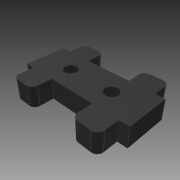
# Autodesk Inventor part: y_carriage_belt_iddler_holder
Saved by Autodesk Inventor 2014 (Build 180170000, 170)
## iProperties
Created: 2013-12-07
Part Number: y_carriage_belt_iddler_holder
Material: Plywood, Finish
Document SubType Name: Modeling
Designer: buben
Density: 0.552 g/cm^3
Appearance: Plywood - New
Author: buben
Subject: Laser Cutted
Autodesk Inventor part; units mm, degrees
ref_plane "YZ Plane" through (0, 0, 0) normal (1, 0, 0) x (0, 1, 0)
ref_plane "XZ Plane" through (0, 0, 0) normal (0, 1, 0) x (-1, 0, 0)
ref_plane "XY Plane" through (0, 0, 0) normal (0, 0, 1) x (1, 0, 0)
sketch "Sketch1" plane through (0, 0, 0) normal (0, 0, 1) x (1, 0, 0)
  line L0 (0, 0) -> (37, 0)
  line L1 (37, 0) -> (37, 13.5)
  line L2 (37, 13.5) -> (0, 13.5)
  line L3 (0, 13.5) -> (0, 0)
  dimension "d0" = 13.5
  dimension "d1" = 37
  constraints: 8 end point, 2 parallel, 1 horizontal, 1 perpendicular
  measures "d0" distance of L2.end L0.start
  measures "d1" distance of L0.start L0.end
extrude "Extrusion1" add sketch "Sketch1" along normal blind 6.5
sketch "Sketch2" plane through (0, 0, 6.5) normal (0, 0, 1) x (1, 0, 0)
  line L0 (0, 0) -> (37, 0) projected
  line L1 (37, 13.5) -> (0, 13.5) projected
  line L2 (3, 13.5) -> (11, 13.5)
  line L3 (11, 13.5) -> (11, 18)
  line L4 (9, 20) -> (5, 20)
  line L5 (3, 18) -> (3, 13.5)
  line L6 (26, 13.5) -> (34, 13.5)
  line L7 (34, 13.5) -> (34, 18)
  line L8 (32, 20) -> (28, 20)
  line L9 (26, 18) -> (26, 13.5)
  line L10 (3, 0) -> (11, 0)
  line L11 (11, 0) -> (11, -4.5)
  line L12 (9, -6.5) -> (5, -6.5)
  line L13 (3, -4.5) -> (3, 0)
  line L14 (26, 0) -> (34, 0)
  line L15 (34, 0) -> (34, -4.5)
  line L16 (32, -6.5) -> (28, -6.5)
  line L17 (26, -4.5) -> (26, 0)
  arc A0 (5, 20) -> (3, 18) centre (5, 18) ccw
  arc A1 (11, 18) -> (9, 20) centre (9, 18) ccw
  arc A2 (28, 20) -> (26, 18) centre (28, 18) ccw
  arc A3 (34, 18) -> (32, 20) centre (32, 18) ccw
  arc A4 (3, -4.5) -> (5, -6.5) centre (5, -4.5) ccw
  arc A5 (9, -6.5) -> (11, -4.5) centre (9, -4.5) ccw
  arc A6 (26, -4.5) -> (28, -6.5) centre (28, -4.5) ccw
  arc A7 (32, -6.5) -> (34, -4.5) centre (32, -4.5) ccw
  line L18 (11, 15.75) -> (26, 15.75) construction
  point P0 (18.5, 15.75)
  point P1 (18.5, 13.5)
  dimension "d4" = 2
  dimension "d5" = 8
  dimension "d6" = 8
  dimension "d7" = 15
  dimension "d8" = 6.5
  dimension "d9" = 6.5
  constraints: 34 end point, 16 point on circle, 16 tangent, 8 centre point, 8 parallel, 7 equal radius, 6 collinear, 5 perpendicular, 4 horizontal, 4 midpoint, 4 point on line, 1 vertical alignment
  measures "d4" radius of A0
  measures "d5" distance between parallel lines of L3 L5
  measures "d6" distance between parallel lines of L7 L9
  measures "d7" distance between parallel lines of L9 L3
  measures "d8" distance between parallel lines of L1 L4
  measures "d9" distance between parallel lines of L12 L0
extrude "Extrusion2" add sketch "Sketch2" against normal blind 6.5
sketch "Sketch3" plane through (0, 0, 6.5) normal (0, 0, 1) x (1, 0, 0)
  line L0 (26, 13.5) -> (11, 13.5) projected
  line L1 (0, 13.5) -> (0, 0) projected
  line L2 (11, 6.75) -> (26, 6.75) construction
  circle A0 centre (11, 6.75) radius 2.25
  circle A1 centre (26, 6.75) radius 2.25
  point P0 (18.5, 6.75)
  point P1 (18.5, 13.5)
  point P2 (0, 6.75)
  dimension "d12" = 4.5
  dimension "d13" = 15
  constraints: 3 midpoint, 2 centre point, 2 coincident, 2 end point, 1 equal radius, 1 horizontal alignment, 1 perpendicular, 1 vertical alignment
  measures "d12" diameter of A1
  measures "d13" distance of L2.start L2.end
extrude "Extrusion3" cut sketch "Sketch3" against normal through all
equation "\"d9\" = d8"
body "Solid1"
